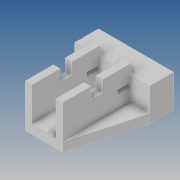
# Autodesk Inventor part: Talon for encoder
Saved by Autodesk Inventor 2019 (Build 230136000, 136)
## iProperties
Created: 2018-01-27
Part Number: Talon for encoder
Material: Generic
Document SubType Name: Modeling
Designer: kalra.rohan
Density: 1 g/cm^3
Appearance: Default
Author: kalra.rohan
Autodesk Inventor part; units mm, degrees
ref_plane "YZ Plane" through (0, 0, 0) normal (1, 0, 0) x (0, 1, 0)
ref_plane "XZ Plane" through (0, 0, 0) normal (0, 1, 0) x (-1, 0, 0)
sketch "Sketch1" plane through (0, 0, 0) normal (0, 0, 1) x (1, 0, 0)
  line L0 (0, 0) -> (3.302, 0)
  line L1 (3.302, 0) -> (3.302, -27.94)
  line L2 (3.302, -27.94) -> (0, -27.94)
  line L3 (0, -27.94) -> (0, 0)
  dimension "d0" = 3.302
  dimension "d1" = 27.94
  constraints: 8 end point, 2 parallel, 1 horizontal, 1 perpendicular
  measures "d0" distance between parallel lines of L1 L3
  measures "d1" distance of L2.end L0.start
extrude "Extrusion1" add sketch "Sketch1" along normal blind 2.54
sketch "Sketch2" plane through (0, 0, 2.54) normal (0, 0, 1) x (1, 0, 0)
  line L0 (3.302, 0) -> (0, 0) projected
  line L1 (0, 0) -> (0, -27.94) projected
  line L2 (0, -27.94) -> (3.302, -27.94) projected
  line L3 (3.302, -27.94) -> (3.302, 0) projected
ref_plane "Work Plane1" through (0, 0, 27.94) normal (0, 0, 1) x (1, 0, 0)
sketch "Sketch3" plane through (0, 0, 27.94) normal (0, 0, 1) x (1, 0, 0)
  line L0 (0, -6.985) -> (3.302, -6.985)
  line L1 (3.302, -6.985) -> (3.302, -20.955)
  line L2 (3.302, -20.955) -> (0, -20.955)
  line L3 (0, -20.955) -> (0, -6.985)
  line L4 (0, -27.94) -> (3.302, -27.94) projected
  line L5 (0, 0) -> (0, -27.94) projected
  dimension "d5" = 3.302
  dimension "d6" = 13.97
  dimension "d7" = 6.985
  dimension "d8" = 0
  constraints: 8 end point, 2 parallel, 1 horizontal, 1 perpendicular
  measures "d5" distance between parallel lines of L3 L1
  measures "d6" distance of L2.end L0.start
  measures "d7" distance between parallel lines of L4 L2
  measures "d8" distance between parallel lines of L5 L3
loft "Loft1" add profiles "Sketch2", "Sketch3"
sketch "Sketch4" plane through (3.302, -27.94, 0) normal (1, 0, 0) x (0, 0, -1)
  line L0 (0, 0) -> (0, 27.94) projected
  line L1 (-2.54, 0) -> (-27.94, 6.985) projected
  line L2 (0, 27.94) -> (-2.54, 27.94)
  line L3 (-2.54, 27.94) -> (-2.54, 0)
  line L4 (-2.54, 0) -> (0, 0)
  line L5 (0, 0) -> (0, 27.94)
  line L6 (-2.54, 27.94) -> (-27.94, 20.955) projected
  line L7 (-27.94, 20.955) -> (-2.54, 20.955)
  line L8 (-2.54, 20.955) -> (-2.54, 18.415)
  line L9 (-2.54, 18.415) -> (-27.94, 18.415)
  line L10 (-27.94, 18.415) -> (-27.94, 20.955)
  line L11 (-27.94, 6.985) -> (-2.54, 6.985)
  line L12 (-2.54, 6.985) -> (-2.54, 9.525)
  line L13 (-2.54, 9.525) -> (-27.94, 9.525)
  line L14 (-27.94, 9.525) -> (-27.94, 6.985)
  dimension "d13" = 2.54
  dimension "d14" = 2.54
  constraints: 24 end point, 6 parallel, 3 horizontal, 3 perpendicular, 2 point on line
  measures "d13" distance of L13.end L1.end
  measures "d14" distance of L9.end L6.end
extrude "Extrusion2" add sketch "Sketch4" along normal blind 8.89 contours L4 L3 L2 L0 | L1 L11 L3 | L14 L13 L3 L11 | L3 L9 L10 L7
sketch "Sketch5" plane through (12.192, -27.94, 0) normal (1, 0, 0) x (0, 0, -1)
  line L0 (-27.94, 20.955) -> (-27.94, 6.985) projected
  line L1 (-27.94, 6.985) -> (-2.54, 6.985)
  line L2 (0, 0) -> (-2.54, 0) projected
  line L3 (-2.54, 0) -> (-2.54, 6.985)
  line L4 (-2.54, 0) -> (-27.94, 6.985) projected
  line L5 (-2.54, 0) -> (-27.94, 6.985)
  point P0 (0, 27.94)
  constraints: 6 end point, 1 collinear, 1 horizontal, 1 vertical
extrude "Extrusion3" cut sketch "Sketch5" against normal blind 8.89
sketch "Sketch6" plane through (12.192, -20.955, 2.54) normal (0, -1, 0) x (1, 0, 0)
  line L0 (-2.286, 5.08) -> (-4.445, 5.08)
  line L1 (-4.445, 5.08) -> (-4.445, 0)
  line L2 (-4.445, 0) -> (-2.286, 0)
  line L3 (-2.286, 0) -> (-2.286, 5.08)
  line L4 (-8.89, 0) -> (0, 0) projected
  line L5 (0, 25.4) -> (0, 0) projected
  point P0 (-12.192, -2.54)
  dimension "d19" = 0
  dimension "d20" = 5.08
  dimension "d21" = 2.286
  dimension "d22" = 2.159
  constraints: 8 end point, 2 parallel, 1 horizontal, 1 perpendicular
  measures "d19" distance between parallel lines of L4 L2
  measures "d20" distance of L0.end L1.end
  measures "d21" distance between parallel lines of L5 L3
  measures "d22" distance of L0.start L0.end
extrude "Extrusion4" cut sketch "Sketch6" against normal blind 25.4
sketch "Sketch7" plane through (12.192, -20.955, 2.54) normal (0, -1, 0) x (1, 0, 0)
  line L0 (0, 14.9225) -> (-0.635, 14.9225)
  line L1 (-0.635, 14.9225) -> (-0.635, 10.4775)
  line L2 (-0.635, 10.4775) -> (0, 10.4775)
  line L3 (0, 10.4775) -> (0, 14.9225)
  line L4 (0, 25.4) -> (0, 0) projected
  line L5 (-8.89, 25.4) -> (0, 25.4) projected
  point P0 (-12.192, -2.54)
  dimension "d25" = 0.635
  dimension "d26" = 4.445
  dimension "d27" = 0
  dimension "d28" = 10.4775
  constraints: 8 end point, 2 parallel, 1 horizontal, 1 perpendicular
  measures "d25" distance of L1.end L2.end
  measures "d26" distance of L2.end L0.start
  measures "d27" distance between parallel lines of L4 L3
  measures "d28" distance between parallel lines of L5 L0
extrude "Extrusion5" cut sketch "Sketch7" against normal blind 25.4
sketch "Sketch8" plane through (12.192, -27.94, 0) normal (1, 0, 0) x (0, 0, -1)
  line L0 (-2.54, 18.415) -> (-2.54, 20.955) projected
  line L1 (-13.0175, 20.955) -> (-13.0175, 18.415) projected
  line L2 (-2.54, 20.955) -> (-13.0175, 20.955)
  line L3 (-13.0175, 20.955) -> (-13.0175, 18.415)
  line L4 (-13.0175, 18.415) -> (-2.54, 18.415)
  line L5 (-2.54, 18.415) -> (-2.54, 20.955)
  line L6 (-2.54, 9.525) -> (-13.0175, 9.525) projected
  line L7 (-27.94, 6.985) -> (-2.54, 6.985) projected
  line L8 (-2.54, 9.525) -> (-13.0175, 9.525)
  line L9 (-13.0175, 9.525) -> (-13.0175, 6.985)
  line L10 (-13.0175, 6.985) -> (-2.54, 6.985)
  line L11 (-2.54, 6.985) -> (-2.54, 9.525)
  line L12 (-17.4625, 20.955) -> (-13.0175, 20.955) projected
  line L13 (-27.94, 9.525) -> (-27.94, 18.415) projected
  line L14 (-17.4625, 20.955) -> (-27.94, 20.955)
  line L15 (-27.94, 20.955) -> (-27.94, 18.415)
  line L16 (-27.94, 18.415) -> (-17.4625, 18.415)
  line L17 (-17.4625, 18.415) -> (-17.4625, 20.955)
  line L18 (-17.4625, 6.985) -> (-17.4625, 9.525) projected
  line L19 (-17.4625, 9.525) -> (-27.94, 9.525)
  line L20 (-27.94, 9.525) -> (-27.94, 6.985)
  line L21 (-27.94, 6.985) -> (-17.4625, 6.985)
  line L22 (-17.4625, 6.985) -> (-17.4625, 9.525)
  point P0 (0, 27.94)
  constraints: 32 end point, 8 parallel, 4 horizontal, 4 perpendicular, 4 point on line
extrude "Extrusion6" add sketch "Sketch8" along normal blind 3.81
sketch "Sketch9" plane through (0, 0, 0) normal (0, 0, -1) x (-1, 0, 0)
  point P0 (0, 0)
sketch "Sketch10" plane through (0, 0, 0) normal (0, 0, -1) x (-1, 0, 0)
  line L0 (-12.192, -27.94) -> (0, -27.94) projected
  line L1 (0, -27.94) -> (0, 0) projected
  line L2 (-12.192, -27.94) -> (0, -27.94)
  line L3 (0, -27.94) -> (0, 0)
  line L4 (0, 0) -> (-12.192, 0)
  line L5 (-12.192, 0) -> (-12.192, -27.94)
  constraints: 8 end point, 2 parallel, 1 horizontal, 1 perpendicular
extrude "Extrusion7" add sketch "Sketch10" along normal blind 6.35
sketch "Sketch13" plane through (12.192, -27.94, 0) normal (1, 0, 0) x (0, 0, -1)
  point P0 (0, 27.94)
sketch "Sketch14" plane through (12.192, -27.94, 0) normal (1, 0, 0) x (0, 0, -1)
  point P0 (0, 27.94)
sketch "Sketch15" plane through (12.192, -27.94, 0) normal (1, 0, 0) x (0, 0, -1)
  circle A0 centre (1.905, 13.97) radius 2.54
  line L0 (6.35, 27.94) -> (6.35, 0) projected
  line L1 (-2.54, 27.94) -> (6.35, 27.94) projected
  point P0 (0, 27.94)
  dimension "d41" = 5.08
  dimension "d42" = 4.445
  dimension "d43" = 13.97
  constraints: 1 centre point
  measures "d41" diameter of A0
  measures "d42" distance from line of A0.centre L0
  measures "d43" distance from line of A0.centre L1
extrude "Extrusion9" cut sketch "Sketch15" against normal blind 254
sketch "Sketch17" plane through (12.192, -27.94, 0) normal (1, 0, 0) x (0, 0, -1)
  circle A0 centre (1.905, 13.97) radius 2.54 projected
  circle A1 centre (1.905, 13.97) radius 2.54
  point P0 (0, 27.94)
  constraints: 2 coincident, 1 centre point, 1 concentric
extrude "Extrusion10" add sketch "Sketch17" against normal blind 12.192
body "Solid1"
